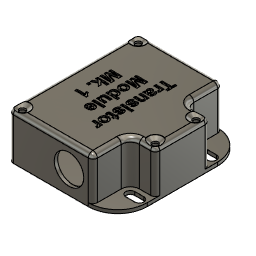
TransisorModuleCase v19 (Autodesk Fusion 360 design; units mm, degrees)
Autodesk Fusion 360 part; units mm, degrees
sketch "Sketch1" plane through (0, 0, 0) normal (0, 1, 0) x (1, 0, 0) in component "ModuleHouse"
  line L0 (0, 0) -> (16, 0)
  line L1 (16, 0) -> (16, -27)
  line L2 (16, -27) -> (0, -27)
  line L3 (0, -27) -> (0, 0)
  line L4 (16, -27) -> (14, -27)
  line L5 (14, -27) -> (14, -17)
  circle A0 centre (14, -17) radius 1.35
  line L6 (0, -27) -> (-1, -27)
  line L7 (-1, -27) -> (-1, -42)
  line L8 (-1, -42) -> (47, -42)
  line L9 (-1, -27) -> (-1, 0)
  line L10 (-1, 0) -> (0, 0)
  line L11 (-1, 0) -> (-1, 15)
  line L12 (-1, 15) -> (47, 15)
  line L13 (47, 15) -> (47, -42)
  line L14 (47, -42) -> (-1, -42)
  line L15 (-1, -42) -> (-1, 15)
  line L16 (-1, -42) -> (0.5, -42)
  line L17 (0.5, -42) -> (0.5, -40.5)
  line L18 (0.5, -40.5) -> (-1, -40.5)
  line L19 (-1, -40.5) -> (-1, -42)
  line L20 (0.5, -40.5) -> (45.5, -40.5)
  line L21 (45.5, -40.5) -> (45.5, 13.5)
  line L22 (45.5, 13.5) -> (0.5, 13.5)
  line L23 (0.5, 13.5) -> (0.5, -40.5)
  line L24 (-1, -42) -> (4, -42)
  line L25 (4, -42) -> (4, -29.5)
  line L26 (4, -29.5) -> (-1, -29.5)
  line L27 (-1, -29.5) -> (-1, -42)
  line L28 (4, -29.5) -> (40, -29.5)
  line L29 (40, -29.5) -> (40, 2.5)
  circle A1 centre (14, -17) radius 5
  circle A2 centre (40, -29.5) radius 5.5
  line L30 (34.5, -29.5) -> (34.5, -40.5)
  line L31 (40, -24) -> (45.5, -24)
  circle A3 centre (40, -29.5) radius 4
  line L32 (40, -25.5) -> (47, -25.5)
  line L33 (36, -29.5) -> (36, -42)
  circle A4 centre (40, 2.5) radius 5.5
  circle A5 centre (40, 2.5) radius 4
  line L34 (40, -1.5) -> (47, -1.5)
  line L35 (40, -3) -> (45.5, -3)
  line L36 (36, 2.5) -> (36, 15)
  line L37 (34.5, 2.5) -> (34.5, 13.5)
  dimension "d1" = 16
  dimension "d2" = 27
  dimension "d3" = 2
  dimension "d4" = 10
  dimension "d5" = 2.7
  dimension "d6" = 1
  dimension "d7" = 15
  dimension "d8" = 48
  dimension "d9" = 15
  dimension "d10" = 1.5
  dimension "d11" = 1.5
  dimension "d12" = 45
  dimension "d13" = 54
  dimension "d16" = 5
  dimension "d17" = 12.5
  dimension "d18" = 36
  dimension "d21" = 32
  dimension "d30" = 10
  dimension "d101" = 11
  dimension "d102" = 8
  dimension "d103" = 8
  constraint horizontal L0
  constraint vertical L1
  constraint horizontal L2
  constraint vertical L3
  constraint coincident L0.start L3.end
  constraint perpendicular L1 L4
  constraint perpendicular L2 L5
  constraint coincident L5.end A0.centre
  constraint perpendicular L3 L6
  constraint perpendicular L6 L7
  constraint perpendicular L7 L8
  constraint perpendicular L0 L9
  constraint perpendicular L9 L10
  constraint perpendicular L10 L11
  constraint horizontal L12
  constraint horizontal L14
  constraint vertical L15
  constraint horizontal L16
  constraint vertical L17
  constraint horizontal L18
  constraint vertical L19
  constraint horizontal L20
  constraint horizontal L22
  constraint vertical L23
  constraint horizontal L24
  constraint vertical L25
  constraint horizontal L26
  constraint vertical L27
  constraint perpendicular L21 L28
  constraint concentric A0 A1
  constraint coincident L28.end L29.start
  constraint coincident A2 L30.start
  constraint coincident L28 L30.start
  constraint coincident L20 L30.end
  constraint tangent A2 L30
  constraint perpendicular L20 L30
  constraint coincident A2 L31.start
  constraint coincident L29 L31.start
  constraint coincident L21 L31.end
  constraint tangent A2 L31
  constraint perpendicular L21 L31
  constraint coincident A3 L32.start
  constraint coincident L29 L32.start
  constraint coincident L13 L32.end
  constraint tangent A3 L32
  constraint perpendicular L13 L32
  constraint coincident A3 L33.start
  constraint coincident L28 L33.start
  constraint coincident L8 L33.end
  constraint tangent A3 L33
  constraint perpendicular L8 L33
  constraint coincident L29.end A4.centre
  constraint tangent L21 A4
  constraint coincident A5 L34.start
  constraint coincident L29 L34.start
  constraint coincident L13 L34.end
  constraint tangent A5 L34
  constraint perpendicular L13 L34
  constraint coincident A4 L35.start
  constraint coincident L29 L35.start
  constraint coincident L21 L35.end
  constraint tangent A4 L35
  constraint coincident A5 L36.start
  constraint coincident L12 L36.end
  constraint tangent A5 L36
  constraint perpendicular L12 L36
  constraint coincident A4 L37.start
  constraint coincident L22 L37.end
  constraint tangent A4 L37
  constraint perpendicular L22 L37
  measures "d1" distance of L0.start L0.end
  measures "d2" distance of L0.start L2.end
  measures "d3" distance of L1.end L4.end
  measures "d4" distance of L4.end L5.end
  measures "d5" diameter of A0
  measures "d6" distance of L2.end L6.end
  measures "d7" distance of L6.end L7.end
  measures "d8" distance of L7.end L8.end
  measures "d9" distance of L9.end L11.end
  measures "d10" distance of L7.end L16.end
  measures "d11" distance of L7.end L18.end
  measures "d12" distance of L17.end L20.end
  measures "d13" distance of L17.end L22.end
  measures "d16" distance of L7.end L24.end
  measures "d17" distance of L7.end L26.end
  measures "d18" distance of L25.end L28.end
  measures "d21" distance of L28.end L29.end
  measures "d30" diameter of A1
  measures "d101" diameter of A2
  measures "d102" diameter of A3
  measures "d103" diameter of A5
extrude "Extrude1" add sketch "Sketch1" against normal blind 1.5 contours L0 L10 L11 L12 L15 L22 L23 L36 | L0 L2 L3 L23 | L3 L6 L9 L10 L15 | L0 L1 L2 L4 L22 L23 L26 L28 L29 A1 A2 A4 L37 | L0 L1 L2 L5 L23 A1 | L2 L6 L7 L15 L23 L26 | L1 A1 | L1 A1 | L22 A4 L36 L37 | L1 L2 L4 L5 A1 | L20 L23 L25 L26 | L7 L15 L18 L23 L26 L27 | L12 L13 L21 L22 L34 L36 | L21 L22 A4 L36 | L29 A4 A5 L36 | L8 L14 L17 L20 L24 L25 | L7 L8 L14 L15 L16 L17 L18 L19 L24 L27 | L20 L25 L28 L30 | A4 A5 L34 L36 | L21 L29 L31 L35 | L29 A4 L34 | L21 A4 L34 L35 | L8 L14 L20 L25 L33 | L28 L29 A2 A3 | L28 A2 L33 | L20 A2 L30 L33 | L13 L21 L32 L34 | L21 A4 L34 | A5 | L29 A2 L32 | L21 A2 L31 L32 | L28 L29 A3 | L28 L29 A3 | A2 A3 L32 L33 | L20 L21 A2 L33 | L8 L13 L14 L20 L21 L32 L33 | L21 A2 L32 | A0 makes body 1 in component "ModuleHouse"
extrude "Extrude2" add sketch "Sketch1" along normal blind 17 separate body contours L0 L10 L11 L12 L15 L22 L23 L36 | L0 L2 L3 L23 | L3 L6 L9 L10 L15 | L2 L6 L7 L15 L23 L26 | L22 A4 L36 L37 | L7 L15 L18 L23 L26 L27 | L29 A4 A5 L36 | L8 L14 L17 L20 L24 L25 | L7 L8 L14 L15 L16 L17 L18 L19 L24 L27 | L29 A4 L34 | L21 A4 L34 L35 | L8 L14 L20 L25 L33 | L28 L29 A2 A3 | L28 A2 L33 | L20 A2 L30 L33 | L13 L21 L32 L34 | L29 A2 L32 | L21 A2 L31 L32 makes body 2 in component "ModuleHouse"
extrude "Extrude4" add sketch "Sketch1" along normal blind 3 contours L1 A1 | L1 A1 bodies 1 in component "ModuleHouse"
sketch "Sketch2" plane through (0, 17, 0) normal (0, 1, 0) x (-1, 0, 0) in component "ModuleHouse"
  arc A0 (-34.5, -2.5) -> (-40, 3) centre (-40, -2.5) ccw
  line L0 (-40, 3) -> (-45.5, 3)
  line L1 (-45.5, 3) -> (-45.5, 24)
  line L2 (-45.5, 24) -> (-40, 24)
  arc A1 (-40, 24) -> (-34.5, 29.5) centre (-40, 29.5) ccw
  line L3 (-34.5, 29.5) -> (-34.5, 40.5)
  line L4 (-34.5, 40.5) -> (-0.5, 40.5)
  line L5 (-0.5, 40.5) -> (-0.5, -13.5)
  line L6 (-0.5, -13.5) -> (-34.5, -13.5)
  line L7 (-34.5, -13.5) -> (-34.5, -2.5)
  arc A2 (-36, -2.5) -> (-40, 1.5) centre (-40, -2.5) ccw
  line L8 (-36, -2.5) -> (-36, -15)
  line L9 (-36, -15) -> (1, -15)
  line L10 (1, -15) -> (1, 42)
  line L11 (1, 42) -> (-36, 42)
  line L12 (-36, 42) -> (-36, 29.5)
  arc A3 (-40, 25.5) -> (-36, 29.5) centre (-40, 29.5) ccw
  line L13 (-40, 25.5) -> (-47, 25.5)
  line L14 (-47, 25.5) -> (-47, 1.5)
  line L15 (-47, 1.5) -> (-40, 1.5)
  line L16 (1, 42) -> (-2, 42)
  line L17 (-2, 42) -> (-2, 39)
  line L18 (-2, 39) -> (1, 39)
  line L19 (1, 39) -> (1, 42)
  line L20 (-47, 25.5) -> (-44, 25.5)
  line L21 (-44, 25.5) -> (-44, 22.5)
  line L22 (-44, 22.5) -> (-47, 22.5)
  line L23 (-47, 22.5) -> (-47, 25.5)
  line L24 (-47, 1.5) -> (-44, 1.5)
  line L25 (-44, 1.5) -> (-44, 4.5)
  line L26 (-44, 4.5) -> (-47, 4.5)
  line L27 (-47, 4.5) -> (-47, 1.5)
  line L28 (1, -15) -> (-2, -15)
  line L29 (-2, -15) -> (-2, -12)
  line L30 (-2, -12) -> (1, -12)
  line L31 (1, -12) -> (1, -15)
  circle A4 centre (-2, -12) radius 1.35
  circle A5 centre (-2, -12) radius 3
  circle A6 centre (-44, 4.5) radius 1.35
  circle A7 centre (-44, 22.5) radius 1.35
  circle A8 centre (-2, 39) radius 1.35
  circle A9 centre (-2, 39) radius 3
  circle A10 centre (-44, 22.5) radius 3
  circle A11 centre (-44, 4.5) radius 3
  dimension "d104" = 3
  dimension "d105" = 3
  dimension "d106" = 3
  dimension "d107" = 3
  dimension "d108" = 3
  dimension "d109" = 3
  dimension "d110" = 3
  dimension "d111" = 3
  dimension "d112" = 2.7
  dimension "d113" = 2.7
  dimension "d114" = 2.7
  dimension "d115" = 2.7
  constraint horizontal L16
  constraint vertical L17
  constraint horizontal L18
  constraint vertical L19
  constraint coincident L10.end L11.start
  constraint horizontal L20
  constraint vertical L21
  constraint horizontal L22
  constraint vertical L23
  constraint coincident L13.end L14.start
  constraint horizontal L24
  constraint vertical L25
  constraint horizontal L26
  constraint vertical L27
  constraint coincident L14.end L15.start
  constraint horizontal L28
  constraint vertical L29
  constraint horizontal L30
  constraint vertical L31
  constraint coincident L9.end L10.start
  constraint coincident L29.end L30.start
  constraint concentric A4 A5
  constraint coincident L28.end A5
  constraint coincident L25.end L26.start
  constraint coincident L21.end L22.start
  constraint coincident L17.end L18.start
  constraint concentric A8 A9
  constraint coincident L16.end A9
  constraint concentric A7 A10
  constraint coincident L22.end A10
  constraint concentric A6 A11
  constraint coincident L26.end A11
  measures "d104" distance of L10.end L16.end
  measures "d105" distance of L10.end L18.end
  measures "d106" distance of L13.end L20.end
  measures "d107" distance of L13.end L22.end
  measures "d108" distance of L14.end L24.end
  measures "d109" distance of L14.end L26.end
  measures "d110" distance of L9.end L28.end
  measures "d111" distance of L9.end L30.end
  measures "d112" diameter of A4
  measures "d113" diameter of A6
  measures "d114" diameter of A7
  measures "d115" diameter of A8
extrude "Extrude6" add sketch "Sketch2" against normal blind 17 contours L0 L1 L25 L26 A6 A11 | L5 L6 L29 L30 A4 A5 | L0 L1 L25 L26 A6 | L5 L6 L29 L30 A4 | L4 L5 L17 L18 A8 A9 | L1 L2 L21 L22 A7 A10 | L4 L5 L17 L18 A8 | L1 L2 L21 L22 A7 bodies 2 1 in component "ModuleHouse"
sketch "Sketch4" plane through (0, 0, 0) normal (0, 1, 0) x (-1, 0, 0) in component "ModuleHouse"
  line L0 (-36, 29.5) -> (-36, 42)
  line L1 (-36, 42) -> (-47, 42)
  line L2 (-47, 42) -> (-47, 25.5)
  line L3 (-47, 25.5) -> (-40, 25.5)
  arc A0 (-40, 25.5) -> (-36, 29.5) centre (-40, 29.5) ccw
  line L4 (-36, -15) -> (-36, -2.5)
  arc A1 (-36, -2.5) -> (-40, 1.5) centre (-40, -2.5) ccw
  line L5 (-40, 1.5) -> (-47, 1.5)
  line L6 (-47, 1.5) -> (-47, -15)
  line L7 (-47, -15) -> (-36, -15)
  circle A2 centre (-40, -2.5) radius 2
  line L8 (-40, -2.5) -> (-44, -2.5)
  circle A3 centre (-44, -2.5) radius 2
  line L9 (-44, -4.5) -> (-40, -4.5)
  line L10 (-40, -4.5) -> (-40, -0.5)
  line L11 (-40, -0.5) -> (-44, -0.5)
  line L12 (-44, -0.5) -> (-44, -4.5)
  circle A4 centre (-40, 29.5) radius 2
  line L13 (-40, 29.5) -> (-44, 29.5)
  circle A5 centre (-44, 29.5) radius 2
  line L14 (-44, 27.5) -> (-40, 27.5)
  line L15 (-40, 27.5) -> (-40, 31.5)
  line L16 (-40, 31.5) -> (-44, 31.5)
  line L17 (-44, 31.5) -> (-44, 27.5)
  dimension "d116" = 4
  dimension "d117" = 4
  dimension "d118" = 4
  dimension "d119" = 4
  dimension "d120" = 4
  dimension "d121" = 4
  constraint concentric A1 A2
  constraint coincident A1.centre A2.centre
  constraint horizontal L8
  constraint coincident L8.end A3.centre
  constraint horizontal L9
  constraint vertical L10
  constraint horizontal L11
  constraint vertical L12
  constraint coincident A2 L10.end
  constraint coincident A3 L9.start
  constraint concentric A0 A4
  constraint coincident A0.centre A4.centre
  constraint horizontal L13
  constraint coincident L13.end A5.centre
  constraint horizontal L14
  constraint vertical L15
  constraint horizontal L16
  constraint vertical L17
  constraint coincident A4 L15.end
  constraint coincident A5 L14.start
  measures "d116" diameter of A2
  measures "d117" distance of A1.centre L8.end
  measures "d118" diameter of A3
  measures "d119" diameter of A4
  measures "d120" distance of A0.centre L13.end
  measures "d121" diameter of A5
extrude "Extrude8" cut sketch "Sketch4" against normal blind 1.5 contours A2 L10 | A2 L8 L10 | A2 A3 L11 | A2 A3 L9 | A2 L8 L10 | L8 A3 L12 | L8 A3 L12 | A3 L12 | A4 L15 | A4 L13 L15 | A4 A5 L16 | A4 A5 L14 | A4 L13 L15 | L13 A5 L17 | L13 A5 L17 | A5 L17 bodies 2 in component "ModuleHouse"
fillet "Fillet1" radius 2 6 edges at (-1, 7.75, -15) (-1, 7.75, 42) (36, 8.5, 42) (47, 8.5, 25.5) (47, 8.5, 1.5) (36, 8.5, -15) on bodies 2 in component "ModuleHouse"
fillet "Fillet2" radius 2 10 edges at (34.5, 8.5, 40.5) (41.4019, 8.5, 24) (45.5, 8.5, 19.9019) (45.5, 8.5, 7.0981) (41.4019, 8.5, 3) (34.5, 8.5, -13.5) (4.5981, 8.5, -13.5) (0.5, 8.5, -9.4019) (0.5, 8.5, 36.4019) (4.5981, 8.5, 40.5) on bodies 2 in component "ModuleHouse"
fillet "Fillet3" radius 2 24 edges at (9.3384, 0, 15.1919) (1.0168, 0, -8.3667) (0.5, 0, 13.5) (1.0168, 0, 35.3667) (4.1213, 0, 36.8787) (5.6333, 0, 39.9832) (19.7375, 0, 40.5) (33.9142, 0, 39.9142) (34.5, 0, 34) (35.8644, 0, 25.8742) (40.464, 0, 23.4472) (41.865, 0, 20.3925) (44.9832, 0, 18.8667) (45.5, 0, 13.5) (44.9832, 0, 8.1333) (41.865, 0, 6.6075) (40.464, 0, 3.5528) (35.8644, 0, 1.1258) (34.5, 0, -7) (33.9142, 0, -12.9142) (19.7375, 0, -13.5) (5.6333, 0, -12.9832) (4.1213, 0, -9.8787) (9.3384, 3, 18.8081) on bodies 2 in component "ModuleHouse"
fillet "Fillet4" radius 13 2 edges at (47, -0.75, 42) (47, -0.75, -15) on bodies 2 in component "ModuleHouse"
sketch "Sketch1 (2)" plane through (0, 0, 42) normal (0, 0, 1) x (1, 0, 0)
  line L0 (34, -1.5) -> (34, 0)
  line L1 (34, 0) -> (34, 17)
  line L2 (34, 17) -> (1, 17)
  line L3 (1, 17) -> (1, -1.5)
  line L4 (1, -1.5) -> (34, -1.5)
  line L5 (34, 8.5) -> (25.5, 8.5)
  circle A0 centre (25.5, 8.5) radius 6.5
  dimension "d128" = 8.5
  dimension "d129" = 13
  constraint midpoint L1 L5.start
  constraint perpendicular L1 L5
  constraint coincident L5.end A0.centre
  measures "d128" distance of L5.start L5.end
  measures "d129" diameter of A0
extrude "Extrude11" cut sketch "Sketch1 (2)" against normal blind 57 contours A0 bodies 2 in component "ModuleHouse"
sketch "Sketch1 (3)" plane through (0, 17, 0) normal (0, 1, 0) x (-1, 0, 0) in component "ModuleHouseLid"
  arc A0 (1, 40) -> (-1, 42) centre (-1, 40) ccw
  line L0 (-1, 42) -> (-34, 42)
  line L1 (-32.5, 40.5) -> (-6.9749, 40.5)
  line L2 (-0.5, 34.0251) -> (-0.5, -7.0251)
  line L3 (-6.9749, -13.5) -> (-32.5, -13.5)
  line L4 (-34, -15) -> (-1, -15)
  arc A1 (-1, -15) -> (1, -13) centre (-1, -13) ccw
  line L5 (1, -13) -> (1, 40)
  line L6 (-47, -14.5) -> (-47, 41.5)
  arc A2 (-36, -13) -> (-34, -15) centre (-34, -13) ccw
  arc A3 (-34, 42) -> (-36, 40) centre (-34, 40) ccw
  line L7 (-36, 40) -> (-36, 29.5)
  arc A4 (-40, 25.5) -> (-36, 29.5) centre (-40, 29.5) ccw
  line L8 (-40, 25.5) -> (-45, 25.5)
  arc A5 (-45, 25.5) -> (-47, 23.5) centre (-45, 23.5) ccw
  line L9 (-47, 23.5) -> (-47, 3.5)
  arc A6 (-47, 3.5) -> (-45, 1.5) centre (-45, 3.5) ccw
  line L10 (-45, 1.5) -> (-40, 1.5)
  arc A7 (-36, -2.5) -> (-40, 1.5) centre (-40, -2.5) ccw
  line L11 (-36, -2.5) -> (-36, -13)
  circle A8 centre (-44, 22.5) radius 1.35
  circle A9 centre (-2, 39) radius 1.35
  circle A10 centre (-44, 4.5) radius 1.35
  circle A11 centre (-2, -12) radius 1.35
  arc A12 (-41.0114, 4.7613) -> (-39.2806, 2.9527) centre (-39.019, 4.9356) ccw
  arc A13 (-41.0114, 4.7613) -> (-43.7, 7.485) centre (-44, 4.5) ccw
  arc A14 (-45.5, 9.4749) -> (-43.7, 7.485) centre (-43.5, 9.4749) ccw
  line L12 (-45.5, 9.4749) -> (-45.5, 17.5251)
  arc A15 (-43.7, 19.515) -> (-45.5, 17.5251) centre (-43.5, 17.5251) ccw
  arc A16 (-43.7, 19.515) -> (-41.0114, 22.2387) centre (-44, 22.5) ccw
  arc A17 (-39.2806, 24.0473) -> (-41.0114, 22.2387) centre (-39.019, 22.0644) ccw
  arc A18 (-39.2806, 24.0473) -> (-34.5, 29.5) centre (-40, 29.5) ccw
  line L13 (-34.5, 29.5) -> (-34.5, 38.5)
  arc A19 (-32.5, 40.5) -> (-34.5, 38.5) centre (-32.5, 38.5) ccw
  arc A20 (-4.985, 38.7) -> (-6.9749, 40.5) centre (-6.9749, 38.5) ccw
  arc A21 (-4.985, 38.7) -> (-2.3, 36.015) centre (-2, 39) ccw
  arc A22 (-0.5, 34.0251) -> (-2.3, 36.015) centre (-2.5, 34.0251) ccw
  arc A23 (-2.3, -9.015) -> (-0.5, -7.0251) centre (-2.5, -7.0251) ccw
  arc A24 (-2.3, -9.015) -> (-4.985, -11.7) centre (-2, -12) ccw
  arc A25 (-6.9749, -13.5) -> (-4.985, -11.7) centre (-6.9749, -11.5) ccw
  arc A26 (-34.5, -11.5) -> (-32.5, -13.5) centre (-32.5, -11.5) ccw
  line L14 (-34.5, -11.5) -> (-34.5, -2.5)
  arc A27 (-34.5, -2.5) -> (-39.2806, 2.9527) centre (-40, -2.5) ccw
extrude "Extrude1'" add sketch "Sketch1 (3)" along normal blind 2 separate body contours A0 L0 L4 A1 L5 L6 A2 A3 L7 A4 L8 A5 L9 A6 L10 A7 L11 | L1 L2 L3 A12 A13 A14 L12 A15 A16 A17 A18 L13 A19 A20 A21 A22 A23 A24 A25 A26 L14 A27 makes body 3 in component "ModuleHouseLid"
fillet "Fillet2'" radius 2 16 edges at (36, 19, 34.75) (37.1716, 19, 26.6716) (42.5, 19, 25.5) (46.4142, 19, 24.9142) (47, 19, 13.5) (46.4142, 19, 2.0858) (42.5, 19, 1.5) (37.1716, 19, 0.3284) (36, 19, -7.75) (35.4142, 19, -14.4142) (17.5, 19, -15) (-0.4142, 19, -14.4142) (-1, 19, 13.5) (-0.4142, 19, 41.4142) (17.5, 19, 42) (35.4142, 19, 41.4142) on bodies 3 in component "ModuleHouseLid"
hole "Hole1" at (44, 19, 22.5) direction (0, -1, 0) diameter 6.5 depth 0.1 tip angle 118 bodies 3 in component "ModuleHouseLid"
hole "Hole2" at (2, 19, 39) direction (0, -1, 0) diameter 6.5 depth 0.1 tip angle 118 bodies 3 in component "ModuleHouseLid"
hole "Hole3" at (2, 19, -12) direction (0, -1, 0) diameter 6.5 depth 0.1 tip angle 118 bodies 3 in component "ModuleHouseLid"
hole "Hole4" at (44, 19, 4.5) direction (0, -1, 0) diameter 6.5 depth 0.1 tip angle 118 bodies 3 in component "ModuleHouseLid"
sketch "Sketch2 (2)" plane through (0, 19, 0) normal (0, 1, 0) x (-1, 0, 0) in component "ModuleHouseLid"
  arc A0 (-40.9077, 3.5) -> (-45, 7.5923) centre (-44, 4.5) ccw
  line L0 (-40.9077, 3.5) -> (-40, 3.5)
  arc A1 (-34, -2.5) -> (-40, 3.5) centre (-40, -2.5) ccw
  line L1 (-34, -2.5) -> (-34, -13)
  line L2 (-34, -13) -> (-5.0923, -13)
  arc A2 (-1, -8.9077) -> (-5.0923, -13) centre (-2, -12) ccw
  line L3 (-1, -8.9077) -> (-1, 35.9077)
  arc A3 (-5.0923, 40) -> (-1, 35.9077) centre (-2, 39) ccw
  line L4 (-5.0923, 40) -> (-34, 40)
  line L5 (-34, 40) -> (-34, 29.5)
  arc A4 (-40, 23.5) -> (-34, 29.5) centre (-40, 29.5) ccw
  line L6 (-40, 23.5) -> (-40.9077, 23.5)
  arc A5 (-45, 19.4077) -> (-40.9077, 23.5) centre (-44, 22.5) ccw
  line L7 (-45, 19.4077) -> (-45, 7.5923)
  line L8 (-1, -2.5) -> (-1, 29.7965) construction
  line L9 (-1, 29.7965) -> (-34, 29.7965) construction
  line L10 (-34, 29.7965) -> (-34, -2.5) construction
  line L11 (-34, -2.5) -> (-1, -2.5) construction
  text T0 "Transistor Module\nMk. 1" font "Arial" height 5 bold align centre middle in box 32.2965 x 33 at (-1, -2.5) x (0, 1) y (-1, 0) spacing 1 kerned
  constraint coincident L3
  constraint coincident A1.start
extrude "Extrude5" cut sketch "Sketch2 (2)" against normal blind 0.5 text T0 bodies 3 in component "ModuleHouseLid"
component "ModuleHouse" placed x (1, 0, 0) y (0, 1, 0) z (0, 0, 1) at (0, 0, 0)
component "ModuleHouseLid" placed x (1, 0, 0) y (0, 1, 0) z (0, 0, 1) at (0, 0, 0) in component "ModuleHouse"
equation "d12 = 46.500 mm - 1.5 mm"
equation "d13 = 65.500 mm - 1.5 mm - 5 mm - 5 mm"
